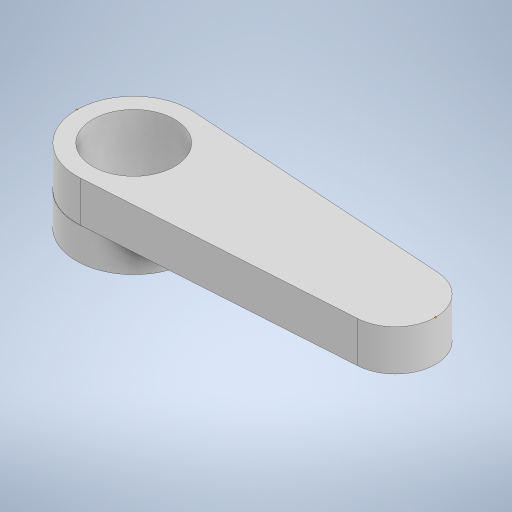
# Autodesk Inventor part: eje de motor
Saved by Autodesk Inventor 2024 (Build 280153000, 153)
## iProperties
Created: 2024-04-28
Part Number: eje de motor
Material: Generic
Document SubType Name: Modeling
Designer: samue
Density: 1 g/cm^3
Appearance: Default
Author: samue
Autodesk Inventor part; units mm, degrees
ref_plane "YZ Plane" through (0, 0, 0) normal (1, 0, 0) x (0, 1, 0)
ref_plane "XZ Plane" through (0, 0, 0) normal (0, 1, 0) x (-1, 0, 0)
sketch "Sketch1" plane through (0, 0, 0) normal (0, 1, 0) x (-1, 0, 0)
  circle A0 centre (0, 0) radius 3.5005
  circle A1 centre (0, 0) radius 2.5
  dimension "d0" = 7.001
  dimension "d1" = 5.0001
  constraints: 2 centre point, 2 coincident
  measures "d0" diameter of A0
  measures "d1" diameter of A1
extrude "Extrusion1" add sketch "Sketch1" along normal blind 2
ref_plane "Work Plane1" through (0, 2, 0) normal (0, 1, 0) x (1, 0, 0)
sketch "Sketch2" plane through (0, 2, 0) normal (0, 1, 0) x (1, 0, 0)
  arc A0 (0.2288, 3.4855) -> (0.2265, -3.4856) centre (0, 0) ccw
  arc A1 (16.1589, -2.4501) -> (16.1605, 2.4395) centre (16, -0.0053) ccw
  circle A2 centre (0, 0) radius 3.5005 projected
  line L0 (0, 3.5005) -> (16.1605, 2.4395)
  line L1 (16.1589, -2.4501) -> (0.2265, -3.4856)
  circle A3 centre (0, 0) radius 2.5 projected
  circle A4 centre (0, 0) radius 2.5
  dimension "d5" = 4.9
  dimension "d6" = 16
  constraints: 4 end point, 4 point on circle, 4 tangent, 3 centre point, 2 coincident, 1 point on line, 1 vertical alignment, 1 other
  measures "d5" diameter of A1
  measures "d6" distance of A1.centre point (0, 0)
extrude "Extrusion2" add sketch "Sketch2" along normal blind 2.5 contours L0 A2 L1 A0 | A0 L1 A2 L0 | L0 A1 L1 A2
body "Solid1"
